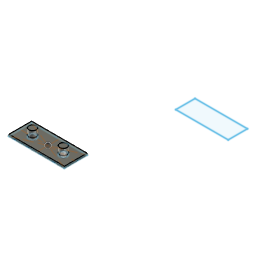
Label v3 (Autodesk Fusion 360 design; units mm, degrees)
Autodesk Fusion 360 part; units mm, degrees
sketch "Schizzo1" plane through (0, 0, 0) normal (0, 0, 1) x (1, 0, 0)
  line L0 (39.554, 71.8617) -> (66.804, 71.8617)
  line L1 (66.804, 71.8617) -> (66.804, 61.8617)
  line L2 (66.804, 61.8617) -> (39.554, 61.8617)
  line L3 (39.554, 61.8617) -> (39.554, 71.8617)
  line L4 (8.0104, 18.4694) -> (37.0104, 18.4694) construction
  line L5 (37.0104, 18.4694) -> (37.0104, 6.4694) construction
  line L6 (37.0104, 6.4694) -> (8.0104, 6.4694) construction
  line L7 (8.0104, 6.4694) -> (8.0104, 18.4694) construction
  line L8 (22.5104, 18.4694) -> (22.5104, 6.4694) construction
  line L9 (8.0104, 12.4694) -> (37.0104, 12.4694) construction
  circle A0 centre (14.5104, 12.4694) radius 1.9
  circle A1 centre (30.5104, 12.4694) radius 1.9
  line L10 (36.9104, 6.5694) -> (8.1104, 6.5694)
  line L11 (8.1104, 6.5694) -> (8.1104, 18.3694)
  line L12 (8.1104, 18.3694) -> (36.9104, 18.3694)
  line L13 (36.9104, 18.3694) -> (36.9104, 6.5694)
  line L14 (36.9104, 6.5694) -> (8.1104, 18.3694) construction
  line L15 (8.1104, 6.5694) -> (36.9104, 18.3694) construction
  point P0 (22.5104, 12.4694)
  dimension "d1" = 27.25
  dimension "d2" = 10
  dimension "d3" = 29
  dimension "d4" = 12
  dimension "d5" = 3.8
  dimension "d6" = 16
  dimension "d7" = 0.1
  dimension "d8" = 0.1
  constraint horizontal L0
  constraint vertical L1
  constraint horizontal L2
  constraint vertical L3
  constraint horizontal L4
  constraint vertical L5
  constraint horizontal L6
  constraint vertical L7
  constraint midpoint L4 L8.start
  constraint midpoint L6 L8.end
  constraint midpoint L7 L9.start
  constraint midpoint L5 L9.end
  constraint coincident L9 A0.centre
  constraint symmetric L8 A0 A1
  constraint horizontal L10
  constraint perpendicular L10 L11
  constraint parallel L10 L12
  constraint parallel L11 L13
  constraint coincident L14 P0
  constraint coincident L15 P0
  constraint midpoint L9 P0
  measures "d1" distance of L1 L3
  measures "d2" distance of L0 L2
  measures "d3" distance of L5 L7
  measures "d4" distance of L4 L6
  measures "d5" diameter of A0
  measures "d6" distance of A0.centre A1.centre
  measures "d7" distance of L4 L12
  measures "d8" distance of L7 L11
extrude "Estrusione1" add sketch "Schizzo1" along normal blind 0.8 contours L10 L11 L12 L13
extrude "Estrusione2" add sketch "Schizzo1" along normal blind 4 contours A0 | A1
equation "d5 = 4 mm - 0.2 mm"
